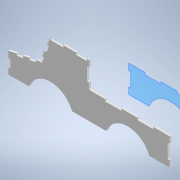
# Autodesk Inventor part: zijplaat
Saved by Autodesk Inventor 2021 (Build 250183000, 183)
## iProperties
Created: 2022-02-01
Part Number: zijplaat
Material: Generic
Document SubType Name: Modeling
Designer: ryan
Density: 1 g/cm^3
Appearance: Default
Author: ryan
Autodesk Inventor part; units mm, degrees
ref_plane "YZ Plane" through (0, 0, 0) normal (1, 0, 0) x (0, 1, 0)
ref_plane "XZ Plane" through (0, 0, 0) normal (0, 1, 0) x (-1, 0, 0)
ref_plane "XY Plane" through (0, 0, 0) normal (0, 0, 1) x (1, 0, 0)
sketch "Sketch1" plane through (0, 0, 0) normal (0, 0, 1) x (1, 0, 0)
  line L0 (0, 0) -> (-250, 0)
  line L1 (-250, 0) -> (-250, 35)
  line L2 (-201.429, 45) -> (-250, 35)
  line L3 (-250, 0) -> (-185, 0)
  line L4 (0, 0) -> (-65, 0)
  line L5 (-185, 85) -> (-201.429, 45)
  line L6 (-185, 0) -> (-185, -10)
  circle A0 centre (-185, -10) radius 36
  line L7 (-65, 0) -> (-65, -10)
  circle A1 centre (-65, -10) radius 36
  line L8 (-250, 0) -> (-250, 3)
  line L9 (-250, 3) -> (0, 3)
  line L10 (0, 0) -> (0, 3)
  line L11 (-250, 35) -> (-250, 25)
  line L12 (-250, 25) -> (-247, 25)
  line L13 (-250, 3) -> (-250, 13)
  line L14 (-250, 13) -> (-247, 13)
  line L15 (-247, 13) -> (-247, 25)
  line L16 (0, 35) -> (-3, 35)
  line L17 (0, 3) -> (0, 13)
  line L18 (0, 13) -> (-3, 13)
  line L19 (-3, 13) -> (-3, 35)
  line L20 (0, 35) -> (0, 45)
  line L21 (0, 45) -> (-125, 45)
  line L22 (-125, 45) -> (-125, 85)
  line L23 (-185, 85) -> (-125, 85)
  line L24 (0, 45) -> (0, 42)
  line L25 (0, 42) -> (-125, 42)
  line L26 (-125, 42) -> (-125, 45)
  line L27 (-125, 45) -> (-100, 45)
  line L28 (-100, 45) -> (-75, 45)
  line L29 (-75, 45) -> (-50, 45)
  line L30 (-50, 45) -> (-25, 45)
  line L31 (-25, 45) -> (0, 45)
  line L32 (-25, 45) -> (-25, 42)
  line L33 (-50, 42) -> (-50, 45)
  line L34 (-75, 42) -> (-75, 45)
  line L35 (-100, 42) -> (-100, 45)
  line L36 (-125, 45) -> (-128, 45)
  line L37 (-128, 45) -> (-128, 85)
  line L38 (-128, 85) -> (-128, 75)
  line L39 (-128, 75) -> (-128, 55)
  line L40 (-128, 75) -> (-125, 75)
  line L41 (-128, 55) -> (-125, 55)
  line L42 (-185, 85) -> (-185, 82)
  line L43 (-185, 82) -> (-128, 82)
  line L44 (-185, 82) -> (-165, 82)
  line L45 (-165, 82) -> (-145, 82)
  line L46 (-145, 82) -> (-128, 82)
  line L47 (-165, 82) -> (-165, 85)
  line L48 (-145, 82) -> (-145, 85)
  line L49 (-185, 85) -> (-185, 38.2522)
  line L50 (-201.429, 45) -> (-198.654, 43.8602)
  line L51 (-198.654, 43.8602) -> (-194.8547, 53.1104)
  line L52 (-194.8547, 53.1104) -> (-191.0554, 62.3605)
  line L53 (-191.0554, 62.3605) -> (-187.2561, 71.6107)
  line L54 (-187.2561, 71.6107) -> (-183.4569, 80.8609)
  line L55 (-194.8547, 53.1104) -> (-197.6298, 54.2502)
  line L56 (-191.0554, 62.3605) -> (-193.8305, 63.5003)
  line L57 (-187.2561, 71.6107) -> (-190.0312, 72.7505)
  line L58 (-183.4569, 80.8609) -> (-186.2319, 82.0006)
  line L59 (-250, 35) -> (-247, 35)
  line L60 (-247, 35) -> (-247, 25)
  line L61 (-250, 35) -> (-250, 32)
  line L62 (-247, 35) -> (-246.5295, 32.7145)
  line L63 (-247, 35) -> (-247.122, 35.5925)
  line L64 (-201.429, 45) -> (-200.8365, 42.122)
  line L65 (-246.5295, 32.7145) -> (-200.8365, 42.122)
  line L66 (-246.5295, 32.7145) -> (-236.7349, 34.7311)
  line L67 (-236.7349, 34.7311) -> (-226.9403, 36.7476)
  line L68 (-226.9403, 36.7476) -> (-217.1458, 38.7642)
  line L69 (-217.1458, 38.7642) -> (-207.3512, 40.7807)
  line L70 (-207.3512, 40.7807) -> (-200.8365, 42.122)
  line L71 (-207.3512, 40.7807) -> (-207.9437, 43.6587)
  line L72 (-217.1458, 38.7642) -> (-217.7383, 41.6422)
  line L73 (-226.9403, 36.7476) -> (-227.5329, 39.6256)
  line L74 (-236.7349, 34.7311) -> (-237.3274, 37.6091)
  point P0 (-218.5708, 3)
  point P1 (-151.4292, 3)
  point P2 (-98.5708, 3)
  point P3 (-31.4292, 3)
  dimension "d0" = 250
  dimension "d1" = 35
  dimension "d6" = 65
  dimension "d8" = 65
  dimension "d11" = 10
  dimension "d12" = 72
  dimension "d13" = 10
  dimension "d14" = 72
  dimension "d15" = 3
  dimension "d18" = 10
  dimension "d19" = 3
  dimension "d20" = 10
  dimension "d22" = 3
  dimension "d23" = 10
  dimension "d24" = 3
  dimension "d35" = 10
  dimension "d36" = 125
  dimension "d37" = 3
  dimension "d38" = 25
  dimension "d39" = 25
  dimension "d40" = 25
  dimension "d41" = 25
  dimension "d42" = 25
  dimension "d43" = 3
  dimension "d44" = 10
  dimension "d45" = 20
  dimension "d46" = 3
  dimension "d47" = 90
  dimension "d48" = 20
  dimension "d49" = 20
  dimension "d50" = 3
  dimension "d51" = 10
  dimension "d52" = 10
  dimension "d53" = 10
  dimension "d54" = 10
  dimension "d55" = 3
  dimension "d56" = 3
  dimension "d57" = 10
  dimension "d58" = 10
  dimension "d59" = 10
  dimension "d60" = 10
  constraints: 150 end point, 41 point on line, 27 perpendicular, 4 vertical, 3 horizontal, 2 centre point, 2 coincident, 2 collinear, 2 parallel
  measures "d0" distance of L0.start L0.end
  measures "d1" distance of L0.end L1.end
  measures "d6" distance of L0.end L3.end
  measures "d8" distance of L0.start L4.end
  measures "d11" distance of L3.end L6.end
  measures "d12" diameter of A0
  measures "d13" distance of L4.end L7.end
  measures "d14" diameter of A1
  measures "d15" distance of L0.end L8.end
  measures "d18" distance of L1.end L11.end
  measures "d19" distance of L11.end L12.end
  measures "d20" distance of L8.end L13.end
  measures "d22" distance of L16.start L16.end
  measures "d23" distance of L9.end L17.end
  measures "d24" distance of L17.end L18.end
  measures "d35" distance of L16.start L20.end
  measures "d36" distance of L20.end L21.end
  measures "d37" distance of L20.end L24.end
  measures "d38" distance of L21.end L27.end
  measures "d39" distance of L27.end L28.end
  measures "d40" distance of L28.end L29.end
  measures "d41" distance of L29.end L30.end
  measures "d42" distance of L30.end L20.end
  measures "d43" distance of L21.end L36.end
  measures "d44" distance of L37.end L38.end
  measures "d45" distance of L38.end L39.end
  measures "d46" distance of L5.start L42.end
  measures "d47" angle of L43 L42
  measures "d48" distance of L42.end L44.end
  measures "d49" distance of L44.end L45.end
  measures "d50" distance of L2.start L50.end
  measures "d51" distance of L50.end L51.end
  measures "d52" distance of L51.end L52.end
  measures "d53" distance of L52.end L53.end
  measures "d54" distance of L53.end L54.end
  measures "d55" distance of L1.end L59.end
  measures "d56" distance of L1.end L61.end
  measures "d57" distance of L62.end L66.end
  measures "d58" distance of L66.end L67.end
  measures "d59" distance of L67.end L68.end
  measures "d60" distance of L68.end L69.end
extrude "Extrusion1" add sketch "Sketch1" against normal blind 3 contours L9 A1 A0 L1 L14 L15 L60 L62 L65 L64 L50 L51 L52 L53 L54 L58 L49 L43 L37 L36 L26 L25 L20 L16 L19 L18 L17 | L25 L32 L21 L20 | L1 L59 L60 L12 | L25 L34 L21 L33 | L2 L63 L59 | L63 L2 L74 L65 L62 | L25 L26 L21 L35 | L36 L37 L41 L22 | L2 L72 L65 L73 | L40 L37 L23 L22 | L2 L64 L65 L71 | L5 L56 L52 L55 | L48 L43 L47 L23 | L5 L58 L49 L54 L57 | L42 L49 L58 L5 | L58 L54 L49
body "Solid1"
